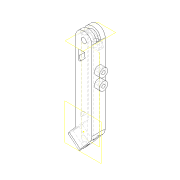
# Autodesk Inventor part: thumb_f1
Saved by Autodesk Inventor 2020.2 (Build 242310000, 310)
## iProperties
Created: 2020-04-08
Part Number: thumb_f1
Material: Generic
Document SubType Name: Modeling
Designer: Bardo91
Density: 1 g/cm^3
Appearance: Default
Author: Bardo91
Autodesk Inventor part; units mm, degrees
ref_plane "YZ Plane" through (0, 0, 0) normal (1, 0, 0) x (0, 1, 0)
ref_plane "XZ Plane" through (0, 0, 0) normal (0, 1, 0) x (-1, 0, 0)
ref_plane "XY Plane" through (0, 0, 0) normal (0, 0, 1) x (1, 0, 0)
sketch "Sketch1" plane through (0, 0, 0) normal (0, 0, 1) x (1, 0, 0)
  line L0 (0, 0) -> (0, 48)
  circle A0 centre (0, 48) radius 1.5
  circle A1 centre (0, 48) radius 5
  circle A2 centre (0, 0) radius 5
  line L1 (-5, 48) -> (-5, 0)
  line L2 (5, 0) -> (5, 48)
  line L3 (-5, 0) -> (5, 0)
  line L4 (-5, 0) -> (-11.4279, -7.6604)
  line L5 (-5, 0) -> (5, 0) construction
  line L6 (-11.4279, -7.6604) -> (-4.6635, -13.3364)
  line L7 (-4.6635, -13.3364) -> (3.8302, -3.2139)
  point P0 (0, 43)
  point P1 (0, 5)
  dimension "d1" = 48
  dimension "d2" = 3
  dimension "d3" = 10
  dimension "d4" = 10
  dimension "d65" = 10
  dimension "d66" = 130
  constraints: 16 end point, 5 point on circle, 4 coincident, 3 centre point, 3 tangent, 2 perpendicular, 2 vertical, 1 equal length, 1 horizontal, 1 parallel
  measures "d1" distance of L0.start L0.end
  measures "d2" diameter of A0
  measures "d3" diameter of A1
  measures "d4" diameter of A2
  measures "d65" distance of L1.end L4.end
  measures "d66" angle of L4 L5
extrude "base" add sketch "Sketch1" along normal blind 8
ref_plane "Work Plane1" through (0, 0, 4) normal (0, 0, 1) x (1, 0, 0)
sketch "Sketch4" plane through (0, 0, 0) normal (0, 1, 0) x (-1, 0, 0)
  line L0 (-1.5, 8.5) -> (1.5, 8.5) projected
  line L1 (0, 8.5) -> (0, -0.4996)
  line L2 (0, 4.0002) -> (-3.5, 4.0002)
  line L3 (0, 4.0002) -> (3.5, 4.0002)
  circle A0 centre (-3.5, 4.0002) radius 1.25
  circle A1 centre (3.5, 4.0002) radius 1.25
  point P0 (0, 0)
  dimension "d20" = 3.5
  dimension "d21" = 3.5
  dimension "thread_hole" = 2.5
  dimension "d23" = 2.5
  constraints: 6 end point, 2 centre point, 2 coincident, 2 horizontal, 2 midpoint, 1 vertical
  measures "d20" distance of L2.start L2.end
  measures "d21" distance of L2.start L3.end
  measures "thread_hole" diameter of A0
  measures "d23" diameter of A1
extrude "thread_hole" cut sketch "Sketch4" along normal through all both and the other way through all contours A0
ref_plane "Work Plane2" through (5, 48, 2) normal (0, 1, 0) x (-1, 0, 0)
sketch "Sketch9" plane through (5, 48, 2) normal (0, 1, 0) x (-1, 0, 0)
  line L0 (5, -2) -> (5, 6)
  line L1 (2, 6) -> (8, 6) projected
  line L2 (5, 2) -> (1.5, 2)
  circle A0 centre (1.5, 2) radius 1.25
  line L3 (1.5, 0.75) -> (0, 0.75)
  line L4 (0, -2) -> (0, 6) projected
  line L5 (1.5, 3.25) -> (0, 3.25)
  point P0 (0, 0)
  point P1 (0, 4)
  dimension "d47" = 3.5
  dimension "d48" = 2.5
  constraints: 8 end point, 2 horizontal, 2 midpoint, 2 point on circle, 2 point on line, 1 centre point, 1 coincident, 1 parallel, 1 tangent
  measures "d47" distance of L2.start L2.end
  measures "d48" diameter of A0
revolve "Revolution2" cut sketch "Sketch9" angle 180 about axis through (0, 48, 0) along (0, 0, 1)
sketch "Sketch10" plane through (-5, 48, 2.75) normal (0, 1, 0) x (1, 0, 0)
  arc A0 (1.5, -2.5) -> (1.5, 0) centre (1.5, -1.25) ccw projected
  circle A1 centre (1.5, -1.25) radius 1.25
  point P0 (5, 2.75)
  point P1 (1.5, 0)
  constraints: 1 coincident, 3 other
extrude "Extrusion8" cut sketch "Sketch10" against normal through all
ref_plane "Work Plane3" through (0, 0, 8.5) normal (0, 0, -1) x (-1, 0, 0)
sketch "Sketch12" plane through (0, 0, 8) normal (0, 0, 1) x (1, 0, 0)
  circle A0 centre (0, 48) radius 1.5 projected
  line L0 (0, 48) -> (0, 42)
  line L1 (0, 42) -> (0, 39)
  line L2 (0, 48) -> (0.7874, 39)
  line L3 (0, 48) -> (9.0344, 48) construction
  line L4 (0.7874, 39) -> (0, 39)
  line L5 (2.25, -5.0972) -> (2.25, 48.0003) projected
  line L6 (0, 42) -> (0.5249, 42)
  point P0 (0, 0)
  dimension "d57" = 6
  dimension "d58" = 3
  dimension "d59" = 85
  constraints: 12 end point, 2 point on line, 1 equal length, 1 horizontal, 1 parallel, 1 perpendicular, 1 vertical
  measures "d57" distance of L0.start L0.end
  measures "d58" distance of L0.end L1.end
  measures "d59" angle of L2 L3
extrude "lock" add sketch "Sketch12" along normal blind 3 contours L6 L2 L4 L1
mirror "Mirror5" about plane through (0, 0, 4) normal (0, 0, 1) of "lock"
chamfer "Chamfer3" distance 3 angle 45 2 edges at (0, 40.5, 8) (0, 40.5, 0)
sketch "Sketch13" plane through (0, 0, 8) normal (0, 0, 1) x (1, 0, 0)
  point P0 (0, 0)
fillet "Fillet5" radius 4 2 edges at (-8.0457, -10.4984, 8) (-8.0457, -10.4984, 0)
sketch "Sketch14" plane through (-5, 0, 8) normal (-0.7660444, 0.6427876, 0) x (0.6427876, 0.7660444, 0)
  arc A0 (-6, 8) -> (-6, 0) centre (-6, 4) ccw projected
  circle A1 centre (-6, 4) radius 1.5
  point P0 (3.2139, 8)
  dimension "d69" = 3
  constraints: 1 centre point, 1 coincident
  measures "d69" diameter of A1
extrude "motor_1" cut sketch "Sketch14" against normal through all
sketch "Sketch15" plane through (5, 0, 0) normal (1, 0, 0) x (0, 0, -1)
  line L0 (-2.75, 48) -> (-5.25, 48) projected
  line L1 (-4, 48) -> (-4, 33)
  line L2 (-4, 33) -> (-4, 26)
  circle A0 centre (-4, 33) radius 2.5
  circle A1 centre (-4, 26) radius 2.5
  point P0 (0, 0)
  dimension "d72" = 15
  dimension "d73" = 7
  dimension "d74" = 5
  dimension "d75" = 5
  constraints: 4 end point, 2 centre point, 2 coincident, 1 midpoint, 1 point on line, 1 vertical
  measures "d72" distance of L1.start L1.end
  measures "d73" distance of L1.end L2.end
  measures "d74" diameter of A0
  measures "d75" diameter of A1
extrude "tensor_1" add sketch "Sketch15" along normal blind 3
sketch "Sketch16" plane through (8, 33, 4) normal (1, 0, 0) x (0, 0, -1)
  circle A0 centre (0, 0) radius 2.5 projected
  circle A1 centre (0, 0) radius 1
  circle A2 centre (0, -7) radius 2.5 projected
  circle A3 centre (0, -7) radius 1
  point P0 (4, -33)
  dimension "d78" = 2
  dimension "d79" = 2
  constraints: 2 centre point, 2 coincident
  measures "d78" diameter of A1
  measures "d79" diameter of A3
extrude "tensor_2" cut sketch "Sketch16" against normal up to surface contours A1 | A3
sketch "Sketch17" plane through (-5, 0, 0) normal (-1, 0, 0) x (0, 0, 1)
  line L0 (0, 0) -> (8, 0) projected
  line L1 (4, 0) -> (4, 5)
  circle A0 centre (4, 5) radius 1.2498
  line L2 (2.7502, -3.6075) -> (2.7502, 48) projected
  dimension "d5" = 8
  dimension "d82" = 5
  constraints: 2 end point, 1 centre point, 1 coincident, 1 midpoint, 1 tangent, 1 vertical
  measures "d82" distance of L1.start L1.end
extrude "Extrusion14" cut sketch "Sketch17" against normal up to surface contours A0
sketch "Sketch7" plane through (0, 0, 8) normal (0, 0, 1) x (1, 0, 0)
  circle A0 centre (0, 48) radius 1.5 projected
  line L0 (0, 48) -> (-1.0419, 53.9088)
  line L1 (0, 48) -> (6, 48) construction
  line L2 (-1.0419, 53.9088) -> (-0.1736, 48.9848)
  line L3 (0, 48) -> (0, 48.9848)
  line L4 (0, 48.9848) -> (-0.1736, 48.9848)
  line L5 (-1.0419, 53.9088) -> (0, 53.9088)
  point P0 (0, 0)
  dimension "d32" = 6
  dimension "d33" = 80
  dimension "d34" = 5
  constraints: 12 end point, 2 perpendicular, 2 point on line, 1 equal length, 1 horizontal, 1 vertical
  measures "d32" distance of L0.start L0.end
  measures "d33" angle of L0 L1
  measures "d34" distance of L0.end L2.end
sketch "Sketch8" plane through (0, 0, 8.5) normal (0, 0, -1) x (-1, 0, 0)
  line L0 (0, 0) -> (0, -5)
  arc A0 (-5, 0) -> (5, 0) centre (0, 0) ccw projected
  line L1 (0, -5) -> (0, -9)
  line L2 (0, -9) -> (-3, -9)
  line L3 (-3, -9) -> (-3, -4)
  dimension "d40" = 4
  dimension "d41" = 3
  constraints: 8 end point, 2 point on circle, 1 horizontal, 1 perpendicular, 1 point on line, 1 vertical
  measures "d40" distance of L0.end L1.end
  measures "d41" distance of L1.end L2.end
equation "\"d23\" = thread_hole"
equation "\"d48\" = thread_hole"
body "Solid1"
